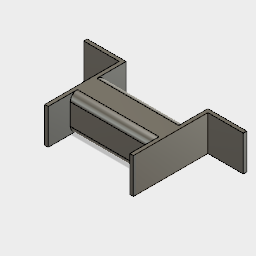
tope_brazo (Autodesk Fusion 360 design; units mm, degrees)
Autodesk Fusion 360 part; units mm, degrees
sketch "Sketch1" plane through (0, 0, 0) normal (0, 1, 0) x (1, 0, 0)
  line L0 (50, 0) -> (50, -15)
  line L1 (0, -15) -> (0, 0)
  line L2 (50, -15) -> (50, -27.5)
  line L3 (50, -27.5) -> (70, -27.5)
  line L4 (70, -27.5) -> (70, -29.5)
  line L5 (70, -29.5) -> (50, -29.5)
  line L6 (50, -29.5) -> (48, -29.5)
  line L7 (48, -29.5) -> (48, -17)
  line L8 (48, -17) -> (2, -17)
  line L9 (2, -17) -> (2, -29.5)
  line L10 (2, -29.5) -> (-20, -29.5)
  line L11 (-20, 14.5) -> (2, 14.5)
  line L12 (2, 14.5) -> (2, 2)
  line L13 (2, 2) -> (48, 2)
  line L14 (48, 2) -> (48, 14.5)
  line L15 (48, 14.5) -> (70, 14.5)
  line L16 (70, 14.5) -> (70, 12.5)
  line L17 (70, 12.5) -> (50, 12.5)
  line L18 (50, 12.5) -> (50, 0)
  line L19 (-20, 14.5) -> (-20, 12.5)
  line L20 (-20, 12.5) -> (0, 12.5)
  line L21 (0, 12.5) -> (0, 0)
  line L22 (-20, -29.5) -> (-20, -27.5)
  line L23 (-20, -27.5) -> (0, -27.5)
  line L24 (0, -27.5) -> (0, -15)
  dimension "d1" = 50
  dimension "d2" = 15
  dimension "d3" = 12.5
  dimension "d4" = 20
  dimension "d5" = 2
  dimension "d6" = 20
  dimension "d7" = 2
  dimension "d8" = 12.5
  dimension "d9" = 46
  dimension "d10" = 12.5
  dimension "d11" = 22
  dimension "d12" = 44
  dimension "d13" = 22
  dimension "d14" = 12.5
  dimension "d15" = 46
  dimension "d16" = 12.5
  dimension "d17" = 22
  dimension "d18" = 2
  dimension "d19" = 20
  dimension "d20" = 2
  dimension "d21" = 20
  dimension "d23" = 2
  measures "d1" distance of L1.end L0.start
  measures "d2" distance of L0.start L0.end
  measures "d3" distance of L0.end L2.end
  measures "d4" distance of L2.end L3.end
  measures "d5" distance of L3.end L4.end
  measures "d6" distance of L4.end L5.end
  measures "d7" distance of L5.end L6.end
  measures "d8" distance of L6.end L7.end
  measures "d9" distance of L7.end L8.end
  measures "d10" distance of L8.end L9.end
  measures "d11" distance of L9.end L10.end
  measures "d12" distance of L10.end L11.start
  measures "d14" distance of L11.end L12.end
  measures "d15" distance of L12.end L13.end
  measures "d16" distance of L13.end L14.end
  measures "d17" distance of L14.end L15.end
  measures "d18" distance of L15.end L16.end
  measures "d19" distance of L16.end L17.end
  measures "d20" distance of L11.start L19.end
  measures "d21" distance of L19.end L20.end
  measures "d23" distance of L10.end L22.end
extrude "Extrude1" add sketch "Sketch1" along normal blind 20
fillet "Fillet1" radius 4 1 edges at (25, 20, 17)
fillet "Fillet2" radius 4 1 edges at (25, 0, 17)
fillet "Fillet3" radius 4 1 edges at (25, 20, -2)
fillet "Fillet4" radius 4 1 edges at (25, 0, -2)
sketch "Sketch2" plane through (50, 0, 0) normal (1, 0, 0) x (0, 0, -1)
  line L0 (-27.5, 0) -> (12.5, 0)
  line L1 (12.5, 0) -> (12.5, 20)
  line L2 (12.5, 20) -> (-27.5, 20)
  line L3 (-27.5, 20) -> (-27.5, 0)
extrude "Extrude2" cut 1 faces at (70, 6.6667, 28.1667) along direction (-1, 0, 0) blind 20
extrude "Extrude3" cut 1 faces at (-20, 6.6667, 28.8333) along direction (1, 0, 0) blind 20
